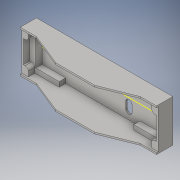
# Autodesk Inventor part: Cam_support
Saved by Autodesk Inventor 2016 (Build 200138000, 138)
## iProperties
Created: 2015-09-25
Part Number: Cam_support
Material: Generic
Document SubType Name: Modeling
Designer: fei
Density: 1 g/cm^3
Appearance: Default
Author: fei
Autodesk Inventor part; units mm, degrees
ref_plane "YZ Plane" through (0, 0, 0) normal (1, 0, 0) x (0, 1, 0)
ref_plane "XZ Plane" through (0, 0, 0) normal (0, 1, 0) x (-1, 0, 0)
ref_plane "XY Plane" through (0, 0, 0) normal (0, 0, 1) x (1, 0, 0)
sketch "Sketch1" plane through (0, 0, 0) normal (0, 0, 1) x (1, 0, 0)
  line L0 (-1066.8, 304.8) -> (1066.8, 304.8)
  line L1 (1066.8, 304.8) -> (1066.8, -304.8)
  line L2 (1066.8, -304.8) -> (-1066.8, -304.8)
  line L3 (-1066.8, -304.8) -> (-1066.8, 304.8)
  point P0 (0, 0)
  point P1 (1066.8, 0)
  point P2 (0, 304.8)
  dimension "d0" = 2133.6
  dimension "d1" = 609.6
  constraints: 8 end point, 2 midpoint, 2 parallel, 1 horizontal, 1 horizontal alignment, 1 perpendicular, 1 vertical alignment
  measures "d0" distance of L0.start L0.end
  measures "d1" distance of L0.end L1.end
extrude "Extrusion1" add sketch "Sketch1" along normal mid plane 25.4
sketch "Sketch3" plane through (0, 0, 12.7) normal (0, 0, 1) x (1, 0, 0)
  line L0 (-1066.8, -304.8) -> (-1066.8, 304.8) projected
  line L1 (1066.8, -304.8) -> (-1066.8, -304.8) projected
  line L2 (-1066.8, 304.8) -> (-1041.4, 304.8)
  line L3 (-1041.4, 304.8) -> (-1041.4, -304.8)
  line L4 (-1041.4, -304.8) -> (-1066.8, -304.8)
  line L5 (-1066.8, -304.8) -> (-1066.8, 304.8)
  line L6 (1066.8, 304.8) -> (1041.4, 304.8)
  line L7 (1041.4, 304.8) -> (1041.4, -304.8)
  line L8 (1041.4, -304.8) -> (1066.8, -304.8)
  line L9 (1066.8, -304.8) -> (1066.8, 304.8)
  point P0 (0, 0)
  dimension "d18" = 25.4
  dimension "d19" = 25.4
  constraints: 16 end point, 4 parallel, 2 horizontal, 2 perpendicular, 2 point on line
  measures "d18" distance of L0.end L2.end
  measures "d19" distance of L6.start L6.end
extrude "Extrusion3" add sketch "Sketch3" along normal blind 203.2
sketch "Sketch5" plane through (0, 0, 0) normal (0, 1, 0) x (-1, 0, 0)
  line L0 (-1041.4, 12.7) -> (1041.4, 12.7) projected
  point P0 (0, 0)
  point P1 (787.4, 12.7)
sketch "Sketch6" plane through (0, 0, 12.7) normal (0, 0, 1) x (1, 0, 0)
  line L0 (-1041.4, 304.8) -> (-1041.4, -304.8) projected
  line L1 (-1041.4, 304.8) -> (-965.2, 304.8)
  line L2 (-965.2, 304.8) -> (-965.2, 177.8)
  line L3 (-965.2, 177.8) -> (-1041.4, 177.8)
  line L4 (-1041.4, 177.8) -> (-1041.4, 304.8)
  line L5 (-1041.4, -304.8) -> (-965.2, -304.8)
  line L6 (-965.2, -304.8) -> (-965.2, -177.8)
  line L7 (-965.2, -177.8) -> (-1041.4, -177.8)
  line L8 (-1041.4, -177.8) -> (-1041.4, -304.8)
  point P0 (0, 0)
  dimension "d30" = 76.2
  dimension "d31" = 127
  dimension "d32" = 127
  dimension "d33" = 76.2
  constraints: 16 end point, 4 parallel, 2 horizontal, 2 perpendicular
  measures "d30" distance of L6.end L7.end
  measures "d31" distance of L5.end L6.end
  measures "d32" distance of L1.end L2.end
  measures "d33" distance of L0.start L1.end
extrude "Extrusion5" add sketch "Sketch6" along normal blind 203.2
mirror "Mirror1" about plane through (0, 0, 0) normal (1, 0, 0) of "Extrusion5"
fillet "Fillet1" radius 50.8 4 edges at (-965.2, 177.8, 114.3) (965.2, 177.8, 114.3) (965.2, -177.8, 114.3) (-965.2, -177.8, 114.3)
sketch "Sketch14" plane through (0, 0, -12.7) normal (0, 0, -1) x (-1, 0, 0)
  line L0 (-1066.8, 304.8) -> (1066.8, 304.8)
  line L1 (1066.8, 304.8) -> (1066.8, 330.2)
  line L2 (1066.8, 330.2) -> (-1066.8, 330.2)
  line L3 (-1066.8, 330.2) -> (-1066.8, 304.8)
  line L4 (1066.8, -304.8) -> (-1066.8, -304.8)
  line L5 (-1066.8, -304.8) -> (-1066.8, -330.2)
  line L6 (-1066.8, -330.2) -> (1066.8, -330.2)
  line L7 (1066.8, -330.2) -> (1066.8, -304.8)
  point P0 (0, 0)
  dimension "d62" = 25.4
  dimension "d63" = 25.4
  constraints: 16 end point, 4 parallel, 2 horizontal, 2 perpendicular, 1 coincident, 1 point on line
  measures "d62" distance of L4.end L5.end
  measures "d63" distance of L0.end L1.end
extrude "Extrusion11" add sketch "Sketch14" against normal blind 228.6
sketch "Sketch15" plane through (-1066.8, 330.2, -12.7) normal (0, 1, 0) x (1, 0, 0)
  line L0 (2133.6, 0) -> (2133.6, -228.6) projected
  line L1 (2133.6, -228.6) -> (2133.6, -254)
  line L2 (2133.6, -254) -> (1879.6, -254)
  line L3 (1879.6, -254) -> (1371.6, -457.2)
  line L4 (1371.6, -457.2) -> (762, -457.2)
  line L5 (762, -457.2) -> (254, -254)
  line L6 (254, -254) -> (0, -254)
  line L7 (0, -254) -> (0, -228.6)
  line L8 (0, -228.6) -> (2133.6, -228.6)
  point P0 (1066.8, -12.7)
  dimension "d66" = 254
  dimension "d67" = 508
  dimension "d68" = 609.6
  dimension "d69" = 508
  dimension "d70" = 254
  dimension "d71" = 228.6
  dimension "d72" = 25.4
  dimension "d73" = 25.4
  constraints: 16 end point, 3 perpendicular, 1 collinear, 1 parallel, 1 vertical
  measures "d66" distance of L1.end L2.end
  measures "d67" horizontal distance of L2.end L3.end
  measures "d68" distance of L3.end L4.end
  measures "d69" horizontal distance of L4.end L5.end
  measures "d70" distance of L5.end L6.end
  measures "d71" distance between parallel lines of L8 L4
  measures "d72" distance of L0.end L1.end
  measures "d73" distance of L6.end L7.end
extrude "Extrusion12" add sketch "Sketch15" against normal blind 25.4
mirror "Mirror4" about plane through (0, 0, 0) normal (0, 1, 0) of "Extrusion12"
sketch "Sketch16" plane through (0, 0, -12.7) normal (0, 0, -1) x (-1, 0, 0)
  line L0 (-457.2, -177.8) -> (-457.2, -76.2)
  line L1 (-355.6, -177.8) -> (-355.6, -76.2)
  arc A0 (-355.6, -76.2) -> (-457.2, -76.2) centre (-406.4, -76.2) ccw
  arc A1 (-457.2, -177.8) -> (-355.6, -177.8) centre (-406.4, -177.8) ccw
  line L2 (-1066.8, 330.2) -> (-1066.8, -330.2) projected
  line L3 (-1066.8, -330.2) -> (1066.8, -330.2) projected
  point P0 (0, 0)
  dimension "d76" = 101.6
  dimension "d77" = 609.6
  dimension "d78" = 152.4
  dimension "d79" = 101.6
  constraints: 4 end point, 4 point on circle, 4 tangent, 2 centre point, 2 vertical
  measures "d76" distance between parallel lines of L0 L1
  measures "d77" distance between parallel lines of L2 L0
  measures "d78" distance from line of L3 A1.centre
  measures "d79" distance of L0.start L0.end
extrude "Extrusion13" cut sketch "Sketch16" against normal blind 25.4
sketch "Sketch20" plane through (0, 0, 12.7) normal (0, 0, 1) x (1, 0, 0)
  line L0 (-965.2, 304.8) -> (-1066.8, 304.8) projected
  line L1 (-1041.4, 304.8) -> (-749.3, 304.8)
  line L2 (-749.3, 304.8) -> (-749.3, 228.6)
  line L3 (-749.3, 228.6) -> (-1041.4, 228.6)
  line L4 (-1041.4, 228.6) -> (-1041.4, 304.8)
  line L5 (-965.2, -304.8) -> (-1028.7, -304.8) projected
  line L6 (-1016, -304.8) -> (-584.2, -304.8)
  line L7 (-584.2, -304.8) -> (-584.2, -228.6)
  line L8 (-584.2, -228.6) -> (-1016, -228.6)
  line L9 (-1016, -228.6) -> (-1016, -304.8)
  point P0 (0, 0)
  dimension "d106" = 431.8
  constraints: 16 end point, 4 parallel, 2 horizontal, 2 perpendicular, 2 point on line
  measures "d106" distance of L7.end L8.end
extrude "Extrusion16" add sketch "Sketch20" along normal blind 101.6
mirror "Mirror5" about plane through (0, 0, 0) normal (1, 0, 0) of "Extrusion16"
sketch "Sketch21" plane through (0, 0, 12.7) normal (0, 0, 1) x (1, 0, 0)
  line L0 (812.8, 304.8) -> (304.8, 304.8) projected
  line L1 (681.4009, 304.8) -> (770.3009, 304.8)
  line L2 (770.3009, 304.8) -> (770.3009, 177.8)
  line L3 (770.3009, 177.8) -> (681.4009, 177.8)
  line L4 (681.4009, 177.8) -> (681.4009, 304.8)
  point P0 (0, 0)
  dimension "d91" = 127
  dimension "d92" = 88.9
  constraints: 8 end point, 2 parallel, 1 horizontal, 1 perpendicular, 1 point on line
  measures "d91" distance of L3.end L1.start
  measures "d92" distance of L2.end L3.end
extrude "Extrusion17" add sketch "Sketch21" along normal blind 101.6
sketch "Sketch22" plane through (0, 0, 12.7) normal (0, 0, 1) x (1, 0, 0)
  line L0 (-812.8, 304.8) -> (-1066.8, 304.8) projected
  line L1 (-812.8, -304.8) -> (-1066.8, -304.8) projected
  line L2 (-1041.4, 304.8) -> (-952.5, 304.8)
  line L3 (-952.5, 304.8) -> (-952.5, -304.8)
  line L4 (-952.5, -304.8) -> (-1041.4, -304.8)
  line L5 (-1041.4, -304.8) -> (-1041.4, 304.8)
  line L6 (-1041.4, -177.8) -> (-1041.4, 177.8) projected
  point P0 (0, 0)
  dimension "d97" = 88.9
  dimension "d98" = 0
  constraints: 8 end point, 2 parallel, 2 point on line, 1 horizontal, 1 perpendicular
  measures "d97" distance between parallel lines of L3 L5
  measures "d98" distance between parallel lines of L6 L5
extrude "Extrusion18" add sketch "Sketch22" along normal blind 101.6
mirror "Mirror7" about plane through (0, 0, 0) normal (1, 0, 0) of "Extrusion18"
sketch "Sketch23" plane through (-1066.8, -330.2, -12.7) normal (0, -1, 0) x (1, 0, 0)
  circle A0 centre (76.2, 76.2) radius 25.4
  line L0 (0, 0) -> (0, 254) projected
  line L1 (2133.6, 0) -> (0, 0) projected
  point P0 (1066.8, 12.7)
  dimension "d101" = 50.8
  dimension "d102" = 76.2
  dimension "d103" = 76.2
  constraints: 1 centre point
  measures "d101" diameter of A0
  measures "d102" distance from line of L0 A0.centre
  measures "d103" distance from line of L1 A0.centre
extrude "Extrusion19" cut sketch "Sketch23" against normal blind 152.4
mirror "Mirror8" about plane through (0, 0, 0) normal (1, 0, 0) of "Extrusion19"
body "Solid1"
